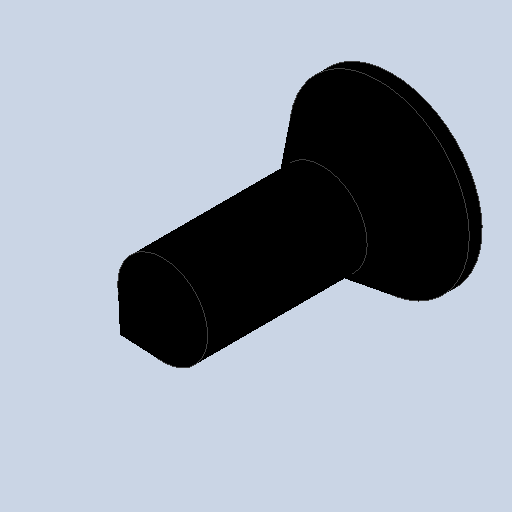
# Autodesk Inventor part: 100031
Saved by Autodesk Inventor 2023 (Build 270158000, 158)
## iProperties
Created: 2023-08-22
Part Number: 100031
Material: Generic
Catalog Web Link: www.cadenas.de
Description: $IDNR.-
Vendor: ROBOTUNITS
Document SubType Name: Modeling
Designer: psAdmin
Manufacturer: ROBOTUNITS
Mass: 1 g
Surface Area: 2.92435 cm^2
Volume: 0.215483 cm^3
Density: 7.85 g/cm^3
Appearance: PSOLRGB-0-0-0
Category: PARTsolutions
Company: ROBOTUNITS
PSOL_IDENT_0: {$CADENAS_DATA/23d-libs/robotunits/pool_bauteile/100031.prj},152 {VTYP=3D},{NB=100031},{LINA=100031}
PSOL_IDENT_1: ,{NN=$IDNR.},{DATE=14.04.2023 08:05:51},{GEOMDATE=20.03.2023 07:40:52},{VERSION=},{LINEID=10},{WBVAR=
PSOL_IDENT_2: },{WBNUMERIC=}  {NB=100031},{LINA=100031},{KT=DUMMY},{IDNR=100031},{GEW=0.001},{ZOLL=73181410}
NB: 100031
NN: $IDNR.
NBSYN: $IDNR.
LINA: 100031
CATALOG: Robotunits
IDNR: 100031
GEW: 0.001
ZOLL: 73181410
SUPPLIER: ROBOTUNITS
ARTICLENO: 100031
BOMINFO: 100031
CREATOR: CADENAS GmbH
Title: 100031
Author: Cadenas PARTsolutions
Autodesk Inventor part; units mm, degrees
sketch "Sketch_1" plane through (0, 0, 0) normal (1, 0, 0) x (0, 1, 0)
  line L0 (0, 0) -> (0, 12.7)
  line L1 (0, 12.7) -> (2.1, 10.7)
  line L2 (2.1, 10.7) -> (2.1, 3.263)
  line L3 (2.1, 3.263) -> (4.2, 0.6)
  line L4 (4.2, 0.6) -> (4.2, 0)
  line L5 (4.2, 0) -> (0, 0)
  line L6 (0, 0) -> (0, 12.7)
  constraints: 14 end point
revolve "Revolution1" add sketch "Sketch_1" angle 360 about axis through (0, 0, 0) along (0, 0, -1)
sketch "Sketch_3" plane through (0, 0, 0) normal (0, 0, -1) x (0, 1, 0)
  line L0 (-2.3, -0.4905) -> (-0.4905, -0.4905)
  line L1 (-0.4905, -0.4905) -> (-0.4905, -2.3)
  line L2 (-0.4905, -2.3) -> (0.4905, -2.3)
  line L3 (0.4905, -2.3) -> (0.4905, -0.4905)
  line L4 (0.4905, -0.4905) -> (2.3, -0.4905)
  line L5 (2.3, -0.4905) -> (2.3, 0.4905)
  line L6 (2.3, 0.4905) -> (0.4905, 0.4905)
  line L7 (0.4905, 0.4905) -> (0.4905, 2.3)
  line L8 (0.4905, 2.3) -> (-0.4905, 2.3)
  line L9 (-0.4905, 2.3) -> (-0.4905, 0.4905)
  line L10 (-0.4905, 0.4905) -> (-2.3, 0.4905)
  line L11 (-2.3, 0.4905) -> (-2.3, -0.4905)
  constraints: 24 end point
extrude "Extrusion1" cut sketch "Sketch_3" against normal blind 2
ref_plane "CS_ANBAU_XY" through (0, 0, 0) normal (0, 0, -1) x (0, 1, 0)
ref_plane "CS_ANBAU_YZ" through (0, 0, 0) normal (0, 1, 0) x (1, 0, 0)
ref_plane "CS_ANBAU_ZX" through (0, 0, 0) normal (1, 0, 0) x (0, 0, -1)
body "Solid1"
